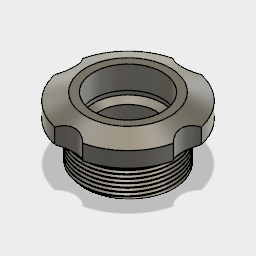
Faucet Toy v7 (Autodesk Fusion 360 design; units mm, degrees)
Autodesk Fusion 360 part; units mm, degrees
cylinder "CylinderPrimitive1" add diameter 24 height 10 placed x (1, 0, 0) y (0, 0, -1) z (0, 1, 0) at (0, 0, 0) makes body 1
thread "Thread1" "ISO Metric profile 24.0 M24x1 6g" major diameter 23.884 minor diameter 22.7375 pitch 1 angle 60 modelled right hand crest width 0.125 on face at (11.9404, 6.6667, 1.1948) crest through (11.942, -0.0625, 0) on bodies 1
hole "Hole1" at (0, 10, 0) direction (0, -1, 0) diameter 18 depth 18 tip angle 118 bodies 1
sketch "Sketch5" plane through (0, 0, 0) normal (0, 1, 0) x (1, 0, 0)
  circle A0 centre (0, 0) radius 16
extrude "Extrude1" add sketch "Sketch5" along normal blind 8 separate body makes body 2
move_body "Move1" bodies 2 to x (1, 0, 0) y (0, 1, 0) z (0, 0, 1) at (0, 8, 0)
hole "Hole2" at (0, 16, 0) direction (0, -1, 0) diameter 18 depth 7 tip angle 118 bodies 2
chamfer "Chamfer1" distance 5 distance2 2 1 edges at (-14.9172, 16, 5.7858) measured on face at (13.5987, 16, 1.0191) on bodies 2
chamfer "Chamfer2" distance 2 distance2 5 1 edges at (-14.9172, 8, 5.7858) measured on face at (15.9205, 10, 1.5931) on bodies 2
cylinder "CylinderPrimitive5" cut diameter 10 height 18 placed x (1, 0, 0) y (0, 0, -1) z (0, 1, 0) at (0, 0, 19) bodies 2
cylinder "CylinderPrimitive6" cut diameter 10 height 18 placed x (1, 0, 0) y (0, 0, -1) z (0, 1, 0) at (19, 0, 0) bodies 2
cylinder "CylinderPrimitive7" cut diameter 10 height 18 placed x (1, 0, 0) y (0, 0, -1) z (0, 1, 0) at (0, 0, -19) bodies 2
cylinder "CylinderPrimitive8" cut diameter 10 height 18 placed x (1, 0, 0) y (0, 0, -1) z (0, 1, 0) at (-19, 0, 0) bodies 2
